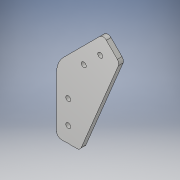
# Autodesk Inventor part: オムニ_固定具1
Saved by Autodesk Inventor 2019.4 (Build 234330000, 330)
## iProperties
Created: 2021-12-02
Part Number: オムニ_固定具1
Material: アルミニウム 6061
Document SubType Name: Modeling
Designer: 堀川皓史
Density: 2.7 g/cm^3
Appearance: アルミニウム - フラット
Author: 堀川皓史
Autodesk Inventor part; units mm, degrees
ref_plane "YZ Plane" through (0, 0, 0) normal (1, 0, 0) x (0, 1, 0)
ref_plane "XZ Plane" through (0, 0, 0) normal (0, 1, 0) x (-1, 0, 0)
ref_plane "XY Plane" through (0, 0, 0) normal (0, 0, 1) x (1, 0, 0)
sketch "スケッチ1" plane through (0, 0, 0) normal (0, 0, 1) x (1, 0, 0)
  line L0 (67.5, 17.5) -> (-67.5, 17.5) construction
  line L1 (-67.5, 17.5) -> (-67.5, -17.5) construction
  line L2 (-67.5, -17.5) -> (67.5, -17.5) construction
  line L3 (67.5, -17.5) -> (67.5, 17.5) construction
  line L4 (67.5, 17.5) -> (-67.5, -17.5) construction
  line L5 (-67.5, 17.5) -> (67.5, -17.5) construction
  circle A0 centre (-60, 35) radius 1.6
  circle A1 centre (-70, 35) radius 1.6
  line L6 (-77.5, 27.5) -> (-53, 27.5)
  line L7 (-53, 27.5) -> (-53, 42.5)
  line L8 (-53, 42.5) -> (-80, 42.5) construction
  line L9 (-77.5, 27.5) -> (-77.5, -27.5)
  line L10 (-77.5, -27.5) -> (-53, -27.5)
  line L11 (-53, -27.5) -> (-53, -42.5)
  line L12 (-53, -42.5) -> (-80, -42.5)
  circle A2 centre (-60, -35) radius 1.6
  circle A3 centre (-70, -35) radius 1.6
  circle A4 centre (-80, -35) radius 1.6
  line L13 (124.2308, -31.7536) -> (484.5935, -392.1164)
  line L14 (484.5935, -392.1164) -> (488.7129, -553.575)
  line L15 (-80, 21.2868) -> (-468.838, -367.5512) construction
  line L16 (-468.838, -367.5512) -> (-479.4446, -356.9446) construction
  line L17 (-479.4446, -356.9446) -> (-90.6066, 31.8934) construction
  line L18 (-90.6066, 31.8934) -> (-80, 21.2868) construction
  line L19 (-80, 42.5) -> (-80, 5.3052) construction
  circle A5 centre (-92.3744, 19.519) radius 1.6
  circle A6 centre (-102.981, 8.9124) radius 1.6
  circle A7 centre (-113.5876, -1.6942) radius 1.6
  line L20 (-92.3744, 19.519) -> (-113.5876, -1.6942) construction
  circle A8 centre (-466.4339, -354.5405) radius 1.6
  circle A9 centre (-455.8273, -343.9339) radius 1.6
  line L21 (-388.4374, -772.2067) -> (-358.1265, -754.7067) construction
  line L22 (-358.1265, -754.7067) -> (-425.6265, -637.7933) construction
  line L23 (-455.9374, -655.2933) -> (-358.1265, -754.7067) construction
  line L24 (-388.4374, -772.2067) -> (-425.6265, -637.7933) construction
  line L25 (-455.9374, -655.2933) -> (-388.4374, -772.2067) construction
  line L26 (-425.6265, -637.7933) -> (-455.9374, -655.2933) construction
  line L27 (455.9374, -655.2933) -> (425.6265, -637.7933) construction
  line L28 (425.6265, -637.7933) -> (358.1265, -754.7067) construction
  line L29 (388.4374, -772.2067) -> (425.6265, -637.7933) construction
  line L30 (455.9374, -655.2933) -> (358.1265, -754.7067) construction
  line L31 (388.4374, -772.2067) -> (455.9374, -655.2933) construction
  line L32 (358.1265, -754.7067) -> (388.4374, -772.2067) construction
  line L33 (0, 0) -> (0, -263.4473) construction
  circle A10 centre (80, -35) radius 1.6
  line L34 (67.5, 17.5) -> (67.5, -17.5) construction
  line L35 (77.5, 27.5) -> (53, 27.5)
  line L36 (77.5, 27.5) -> (77.5, -27.5)
  line L37 (77.5, -27.5) -> (53, -27.5)
  circle A11 centre (60, -35) radius 1.6
  circle A12 centre (70, -35) radius 1.6
  line L38 (53, -27.5) -> (53, -42.5)
  line L39 (53, -42.5) -> (80, -42.5)
  circle A13 centre (60, 35) radius 1.6
  circle A14 centre (70, 35) radius 1.6
  line L40 (80, 42.5) -> (80, 5.3052) construction
  line L41 (53, 42.5) -> (80, 42.5)
  line L42 (53, 27.5) -> (53, 42.5)
  line L43 (-392.0976, -785.867) -> (-404.3476, -764.6493)
  line L44 (-388.4374, -772.2067) -> (-358.1265, -754.7067) construction
  line L45 (-392.0976, -785.867) -> (-344.4662, -758.367)
  circle A15 centre (-336.7211, -756.782) radius 1.6
  circle A16 centre (-341.7211, -748.1218) radius 1.6
  line L46 (-343.7259, -729.6493) -> (-330.2259, -753.032)
  circle A17 centre (-346.7211, -739.4615) radius 1.6
  line L47 (-356.7162, -737.1493) -> (-343.7259, -729.6493)
  line L48 (-344.4662, -758.367) -> (-356.7162, -737.1493)
  circle A18 centre (-407.3428, -774.4615) radius 1.6
  circle A19 centre (-402.3428, -783.1218) radius 1.6
  line L49 (-404.3476, -764.6493) -> (-417.338, -772.1493)
  line L50 (-417.338, -772.1493) -> (-403.838, -795.532)
  line L51 (-403.838, -795.532) -> (-371.6264, -776.9346) construction
  line L52 (-425.6265, -637.7933) -> (-455.9374, -655.2933) construction
  line L53 (-409.7162, -645.3507) -> (-396.7259, -637.8507)
  circle A20 centre (-406.7211, -635.5385) radius 1.6
  line L54 (-455.9374, -655.2933) -> (-425.6265, -637.7933) construction
  circle A21 centre (-411.7211, -626.8782) radius 1.6
  line L55 (-469.5976, -651.633) -> (-421.9662, -624.133)
  line L56 (-421.9662, -624.133) -> (-409.7162, -645.3507)
  line L57 (-396.7259, -637.8507) -> (-410.2259, -614.468)
  circle A22 centre (-416.7211, -618.218) radius 1.6
  line L58 (-469.5976, -651.633) -> (-457.3476, -672.8507)
  circle A23 centre (-467.3428, -670.5385) radius 1.6
  circle A24 centre (-472.3428, -661.8782) radius 1.6
  line L59 (-483.838, -656.968) -> (-451.6264, -638.3706) construction
  line L60 (-470.338, -680.3507) -> (-483.838, -656.968)
  line L61 (-457.3476, -672.8507) -> (-470.338, -680.3507)
  line L62 (469.5976, -651.633) -> (457.3476, -672.8507)
  line L63 (455.9374, -655.2933) -> (425.6265, -637.7933) construction
  line L64 (469.5976, -651.633) -> (421.9662, -624.133)
  circle A25 centre (416.7211, -618.218) radius 1.6
  circle A26 centre (411.7211, -626.8782) radius 1.6
  line L65 (396.7259, -637.8507) -> (410.2259, -614.468)
  circle A27 centre (406.7211, -635.5385) radius 1.6
  line L66 (409.7162, -645.3507) -> (396.7259, -637.8507)
  line L67 (421.9662, -624.133) -> (409.7162, -645.3507)
  circle A28 centre (467.3428, -670.5385) radius 1.6
  circle A29 centre (472.3428, -661.8782) radius 1.6
  line L68 (457.3476, -672.8507) -> (470.338, -680.3507)
  line L69 (470.338, -680.3507) -> (483.838, -656.968)
  line L70 (483.838, -656.968) -> (451.6264, -638.3706) construction
  line L71 (358.1265, -754.7067) -> (388.4374, -772.2067) construction
  line L72 (356.7162, -737.1493) -> (343.7259, -729.6493)
  circle A30 centre (346.7211, -739.4615) radius 1.6
  line L73 (388.4374, -772.2067) -> (358.1265, -754.7067) construction
  circle A31 centre (341.7211, -748.1218) radius 1.6
  line L74 (392.0976, -785.867) -> (344.4662, -758.367)
  line L75 (344.4662, -758.367) -> (356.7162, -737.1493)
  line L76 (343.7259, -729.6493) -> (330.2259, -753.032)
  circle A32 centre (336.7211, -756.782) radius 1.6
  line L77 (392.0976, -785.867) -> (404.3476, -764.6493)
  circle A33 centre (407.3428, -774.4615) radius 1.6
  circle A34 centre (402.3428, -783.1218) radius 1.6
  line L78 (403.838, -795.532) -> (371.6264, -776.9346) construction
  line L79 (417.338, -772.1493) -> (403.838, -795.532)
  line L80 (404.3476, -764.6493) -> (417.338, -772.1493)
  line L81 (-483.838, -367.5512) -> (-468.838, -367.5512) construction
  line L82 (-468.838, -367.5512) -> (-468.838, -648.3077) construction
  line L83 (-468.838, -648.3077) -> (-483.838, -648.3077)
  line L84 (-483.838, -648.3077) -> (-483.838, -367.5512) construction
  line L85 (-283.2277, -604.4352) -> (-262.2277, -640.8083) construction
  line L86 (345.2492, -497.0108) -> (305.7786, -565.3759) construction
  line L87 (265.1134, -631.6538) -> (-234.8866, -631.6538) construction
  line L88 (-234.8866, -631.6538) -> (-234.8866, -1131.6538) construction
  line L89 (-234.8866, -1131.6538) -> (265.1134, -1131.6538) construction
  line L90 (265.1134, -1131.6538) -> (265.1134, -631.6538) construction
  line L91 (265.1134, -631.6538) -> (-234.8866, -1131.6538) construction
  line L92 (-234.8866, -631.6538) -> (265.1134, -1131.6538) construction
  line L93 (-12.841, -157.5) -> (15.1134, -157.5) construction
  circle A35 centre (1.1362, -409.4569) radius 212.5 construction
  line L94 (501.1362, 53.616) -> (-498.8638, 53.616) construction
  line L95 (-498.8638, 53.616) -> (-498.8638, -946.384) construction
  line L96 (-498.8638, -946.384) -> (501.1362, -946.384) construction
  line L97 (501.1362, -946.384) -> (501.1362, 53.616) construction
  line L98 (501.1362, 53.616) -> (-498.8638, -946.384) construction
  line L99 (-498.8638, 53.616) -> (501.1362, -946.384) construction
  circle A36 centre (1.1362, -409.4569) radius 250 construction
  line L100 (-80, 42.5) -> (-90.6066, 31.8934) construction
  line L101 (-80, 42.5) -> (-118.8909, 3.6091)
  line L102 (-118.8909, -6.9975) -> (-113.5876, -12.3008)
  line L103 (-113.5876, -12.3008) -> (-85.2767, -40.3298)
  arc A37 (-118.8909, 3.6091) -> (-118.8909, -6.9975) centre (-113.5876, -1.6942) ccw
  arc A38 (-85.2767, -40.3298) -> (-80, -42.5) centre (-80, -35) ccw
  line L104 (-80, 42.5) -> (-53, 42.5)
  line L105 (-466.4339, -354.5405) -> (-455.8273, -343.9339) construction
  circle A39 centre (-476.338, -638.3077) radius 1.6
  circle A40 centre (-476.338, -623.3077) radius 1.6
  circle A41 centre (-476.338, -378.3077) radius 1.6
  circle A42 centre (-476.338, -393.3077) radius 1.6
  line L106 (-454.0595, -331.5595) -> (-443.4529, -342.1661)
  line L107 (-468.838, -403.3077) -> (-475.5897, -403.3077)
  line L108 (-483.838, -403.3077) -> (-483.838, -367.5512)
  line L109 (-454.0595, -331.5595) -> (-479.4446, -356.9446)
  arc A43 (-479.4446, -356.9446) -> (-483.838, -367.5512) centre (-468.838, -367.5512) ccw
  line L110 (-443.4529, -342.1661) -> (-468.838, -403.3077)
  arc A44 (-475.5897, -403.3077) -> (-477.0864, -403.3077) centre (-476.338, -404.6077) ccw
  line L111 (-475.5897, -403.3077) -> (-477.0864, -403.3077) construction
  line L112 (-477.0864, -403.3077) -> (-483.838, -403.3077)
  point P0 (0, -470)
  point P1 (-102.981, 8.9124)
  point P2 (-77.5, 0)
  point P3 (-407.0319, -705)
  point P4 (-407.0319, -705)
  point P5 (407.0319, -705)
  point P6 (407.0319, -705)
  point P7 (77.5, 0)
  point P8 (-368.2819, -772.117)
  point P9 (-385.4668, -784.9254)
  point P10 (-445.7819, -637.883)
  point P11 (445.7819, -637.883)
  point P12 (465.4668, -646.3614)
  point P13 (368.2819, -772.117)
  point P14 (15.1134, -881.6538)
  point P15 (1.1362, -446.384)
  point P16 (-124.1942, -1.6942)
  point P17 (-476.338, -648.3077)
  point P18 (-476.338, -367.5512)
  dimension "d4" = 135
  dimension "d5" = 35
  dimension "d6" = 3.2
  dimension "d7" = 3.2
  dimension "d8" = 10
  dimension "d9" = 15
  dimension "d10" = 10
  dimension "d11" = 7.5
  dimension "d12" = 7
  dimension "d13" = 70
  dimension "d14" = 3.2
  dimension "d15" = 3.2
  dimension "d16" = 3.2
  dimension "d17" = 10
  dimension "d18" = 10
  dimension "d19" = 7
  dimension "d20" = 15
  dimension "d21" = 7.5
  dimension "d22" = 10
  dimension "d23" = 10
  dimension "d24" = 135
  dimension "d25" = 15
  dimension "d26" = 10
  dimension "d27" = 3.2
  dimension "d28" = 3.2
  dimension "d29" = 3.2
  dimension "d30" = 10
  dimension "d31" = 15
  dimension "d32" = 15
  dimension "d33" = 7.5
  dimension "d34" = 45
  dimension "d35" = 3.2
  dimension "d36" = 3.2
  dimension "d37" = 360
  dimension "d38" = 360
  dimension "d39" = 470
  dimension "d40" = 15
  dimension "d41" = 200
  dimension "d42" = 200
  dimension "d43" = 500
  dimension "d44" = 500
  dimension "d45" = 200
  dimension "d46" = 425
  dimension "d47" = 1000
  dimension "d48" = 1000
  dimension "d49" = 42
  dimension "d50" = 500
  dimension "d51" = 7.5
  dimension "d52" = 7.5
  dimension "d53" = 7.5
  dimension "d54" = 484
  dimension "d55" = 15
  dimension "d56" = 3.2
  dimension "d57" = 3.2
  dimension "d58" = 10
  dimension "d59" = 15
  dimension "d60" = 3.2
  dimension "d61" = 3.2
  dimension "d62" = 15
  dimension "d63" = 230
  dimension "d64" = 10
  dimension "d65" = 10
  dimension "d69" = 3
  dimension "d70" = 1.3
  constraints: 226 end point, 45 centre point, 16 midpoint, 16 symmetric about line, 15 perpendicular, 14 parallel, 13 point on line, 8 coincident, 8 point on circle, 8 vertical alignment, 7 horizontal, 5 tangent, 3 horizontal alignment, 3 vertical, 2 collinear, 242 other
  measures "d4" distance of L2.end L1.end
  measures "d5" distance of L1.end L0.end
  measures "d6" diameter of A0
  measures "d7" diameter of A1
  measures "d8" distance of A0.centre A1.centre
  measures "d9" distance between parallel lines of L6 L8
  measures "d10" distance between parallel lines of L0 L6
  measures "d11" distance from line of L6 A0.centre
  measures "d12" distance from line of L7 A0.centre
  measures "d13" horizontal distance of A1.centre point (0, 0)
  measures "d14" diameter of A2
  measures "d15" diameter of A3
  measures "d16" diameter of A4
  measures "d17" distance of A3.centre A4.centre
  measures "d18" distance of A2.centre A3.centre
  measures "d19" distance from line of L11 A2.centre
  measures "d20" distance between parallel lines of L12 L10
  measures "d21" distance from line of L12 A2.centre
  measures "d22" distance between parallel lines of L10 L2
  measures "d23" distance between parallel lines of L9 L1
  measures "d24" angle of L2 L13
  measures "d25" distance of L15.end L16.end
  measures "d26" distance from line of A1.centre L19
  measures "d27" diameter of A5
  measures "d28" diameter of A6
  measures "d29" diameter of A7
  measures "d30" distance from line of L18 L20.start
  measures "d31" distance of A6.centre L20.start
  measures "d32" distance of L20.end A6.centre
  measures "d33" distance between parallel lines of L15 L20
  measures "d34" angle of L9 L15
  measures "d35" diameter of A8
  measures "d36" diameter of A9
  measures "d39" distance of point (0, -470) point (-407.032, -705)
  measures "d40" distance of L82.end L83.end
  measures "d41" distance between parallel lines of L50 L85
  measures "d42" distance between parallel lines of L79 L86
  measures "d43" distance of L89.end L88.end
  measures "d44" distance of L88.end L87.end
  measures "d45" distance from line of L93.end L8
  measures "d46" diameter of A35
  measures "d47" distance of L96.end L95.end
  measures "d48" distance of L95.end L94.end
  measures "d49" distance of L85.start L85.end
  measures "d50" diameter of A36
  measures "d51" distance from line of L102 L20.end
  measures "d52" radius of A37
  measures "d53" distance between parallel lines of L15 L105
  measures "d54" distance of L20.end L105.end
  measures "d55" distance of L105.end L105.start
  measures "d56" diameter of A39
  measures "d57" diameter of A40
  measures "d58" distance from line of L83 A39.centre
  measures "d59" distance of A40.centre A39.centre
  measures "d60" diameter of A41
  measures "d61" diameter of A42
  measures "d62" distance of A42.centre A41.centre
  measures "d63" distance of A40.centre A42.centre
  measures "d64" distance from line of L105.end L106
  measures "d65" distance from line of L107 A42.centre
  measures "d69" diameter of A44
  measures "d70" distance from line of L107 A44.centre
extrude "押し出し1" add sketch "スケッチ1" along normal blind 3 contours L106 L110 L107 A44 L112 L108 A43 L109
fillet "フィレット1" radius 3 4 edges at (-454.0595, -331.5595, 1.5) (-443.4529, -342.1661, 1.5) (-468.838, -403.3077, 1.5) (-483.838, -403.3077, 1.5)
